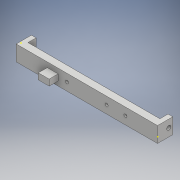
# Autodesk Inventor part: mtv_axelHolder(brakingAxel)3-12
Saved by Autodesk Inventor 2018 (Build 220112000, 112)
## iProperties
Created: 2019-03-12
Part Number: mtv_axelHolder(brakingAxel)3-12
Material: Generic
Document SubType Name: Sheet Metal
Designer: Aditya Kendre
Density: 1 g/cm^3
Sheet Metal Rule: Default_mm
Appearance: Default
Author: Aditya Kendre
Autodesk Inventor part; units mm, degrees
ref_plane "YZ Plane" through (0, 0, 0) normal (1, 0, 0) x (0, 1, 0)
ref_plane "XZ Plane" through (0, 0, 0) normal (0, 1, 0) x (-1, 0, 0)
ref_plane "XY Plane" through (0, 0, 0) normal (0, 0, 1) x (1, 0, 0)
sketch "Sketch1" plane through (0, 0, 0) normal (0, 1, 0) x (-1, 0, 0)
  line L0 (0, 0) -> (150, 0)
  line L1 (150, 0) -> (150, -19.925)
  line L2 (150, -19.925) -> (0, -19.925)
  line L3 (0, -19.925) -> (0, 0)
  dimension "d0" = 150
  dimension "d1" = 19.925
  constraints: 8 end point, 2 parallel, 1 horizontal, 1 perpendicular
  measures "d0" distance of L1.end L2.end
  measures "d1" distance of L0.end L1.end
extrude "Extrusion1" add sketch "Sketch1" along normal blind 4
sketch "Sketch2" plane through (0, 4, 0) normal (0, 1, 0) x (1, 0, 0)
  line L0 (-150, 0) -> (0, 0) projected
  line L1 (0, 19.925) -> (-150, 19.925) projected
  line L2 (0, 0) -> (-5, 0)
  line L3 (-5, 0) -> (-5, 19.925)
  line L4 (-5, 19.925) -> (0, 19.925)
  line L5 (0, 19.925) -> (0, 0)
  line L6 (-150.0001, 0) -> (-145.0001, 0)
  line L7 (-145.0001, 0) -> (-145.0001, 19.925)
  line L8 (-145.0001, 19.925) -> (-150.0001, 19.925)
  line L9 (-150.0001, 19.925) -> (-150.0001, 0)
  dimension "d4" = 5
  dimension "d5" = 5
  constraints: 16 end point, 4 parallel, 3 point on line, 2 horizontal, 2 perpendicular
  measures "d4" distance of L3.end L4.end
  measures "d5" distance of L8.end L7.end
extrude "Extrusion2" add sketch "Sketch2" along normal blind 12.175 contours L9 L1 L7 L0 | L3 L1 L5 L0
sketch "Sketch3" plane through (0, 4, 0) normal (0, 1, 0) x (1, 0, 0)
  line L0 (0, 19.925) -> (0, 0) projected
  line L1 (-150, 0) -> (-150, 19.925) projected
  line L2 (0, 19.925) -> (-150, 19.925)
  line L3 (-150, 19.925) -> (-150, 16.725)
  line L4 (-150, 16.725) -> (0, 16.725)
  line L5 (0, 16.725) -> (0, 19.925)
  dimension "d8" = 3.2
  constraints: 8 end point, 2 parallel, 1 horizontal, 1 perpendicular, 1 point on line
  measures "d8" distance of L3.end L2.end
extrude "Extrusion3" add sketch "Sketch3" along normal blind 4.65
sketch "Sketch4" plane through (0, 4, 0) normal (0, 1, 0) x (1, 0, 0)
  line L0 (-5, 16.725) -> (-145.0001, 16.725) construction
  line L1 (-145.0001, 0) -> (-145.0001, 19.925) construction
  line L2 (-5, 16.725) -> (-145.0001, 16.725) construction
  line L3 (-145.0001, 16.725) -> (-145.0001, 6.225) construction
  line L4 (-145.0001, 6.225) -> (-5, 6.225) construction
  line L5 (-5, 6.225) -> (-5, 16.725) construction
  line L6 (-5, 19.925) -> (-5, 0) projected
  line L7 (-145.0001, 6.225) -> (-5, 6.225)
  line L8 (-5, 6.225) -> (-5, 3.475)
  line L9 (-5, 3.475) -> (-145.0001, 3.475)
  line L10 (-145.0001, 3.475) -> (-145.0001, 6.225)
  point P0 (0, 0)
  dimension "d11" = 10.5
  dimension "d12" = 2.75
  constraints: 16 end point, 4 parallel, 2 horizontal, 2 perpendicular, 2 point on line
  measures "d11" distance of L3.end L2.end
  measures "d12" distance of L7.end L8.end
extrude "Extrusion4" add sketch "Sketch4" along normal blind 3.5
sketch "Sketch5" plane through (-145.0001, 4, 0) normal (1, 0, 0) x (0, 0, -1)
  point P0 (0, -4)
sketch "Sketch6" plane through (-145.0001, 4, 0) normal (1, 0, 0) x (0, 0, -1)
  line L0 (6.225, 0) -> (16.725, 0) construction
  line L1 (16.725, 0) -> (16.725, -7.95) construction
  line L2 (16.725, -7.95) -> (6.225, -7.95) construction
  line L3 (6.225, -7.95) -> (6.225, 0) construction
  line L4 (6.225, 0) -> (16.725, 0) construction
  line L5 (16.725, 0) -> (16.725, 7.95) construction
  line L6 (16.725, 7.95) -> (6.225, 7.95) construction
  line L7 (6.225, 7.95) -> (6.225, 0) construction
  circle A0 centre (11.475, 7.95) radius 2.25
  point P0 (0, -4)
  dimension "d15" = 7.95
  dimension "d16" = 7.95
  dimension "d17" = 4.5
  constraints: 16 end point, 4 parallel, 2 horizontal, 2 perpendicular, 1 centre point, 1 coincident, 1 midpoint, 1 point on line
  measures "d15" distance of L0.end L1.end
  measures "d16" distance of L5.end L4.end
  measures "d17" diameter of A0
extrude "Extrusion5" cut sketch "Sketch6" along normal blind 155.75 and the other way blind 5.75
sketch "Sketch7" plane through (0, 4, 0) normal (0, 1, 0) x (1, 0, 0)
  line L0 (-145.0001, 3.475) -> (-145.0001, 0) projected
  line L1 (-145.0001, 3.475) -> (1.5965, 3.475)
  line L2 (1.5965, 3.475) -> (1.5965, -1.1679)
  line L3 (1.5965, -1.1679) -> (-145.0001, -1.1679)
  line L4 (-145.0001, -1.1679) -> (-145.0001, 3.475)
  line L5 (-145.0001, 3.475) -> (-5, 3.475) projected
  line L6 (-145.0001, 3.475) -> (-155.2913, 3.475)
  line L7 (-155.2913, 3.475) -> (-155.2913, -7.4286)
  line L8 (-155.2913, -7.4286) -> (-145.0001, -7.4286)
  line L9 (-145.0001, -7.4286) -> (-145.0001, 3.475)
  point P0 (0, 0)
  constraints: 16 end point, 4 parallel, 2 horizontal, 2 perpendicular
extrude "Extrusion6" cut sketch "Sketch7" along normal blind 21 and the other way blind 34.875
sketch "Sketch8" plane through (0, 8.65, 0) normal (0, 1, 0) x (1, 0, 0)
  line L0 (-145.0001, 16.725) -> (-145.0001, 19.925) construction
  line L1 (-5, 16.725) -> (-145.0001, 16.725) construction
  line L2 (-145.0001, 19.925) -> (-5, 19.925) construction
  line L3 (-5, 19.925) -> (-5, 16.725) construction
  line L4 (-5, 16.725) -> (-145.0001, 16.725) construction
  line L5 (-145.0001, 16.725) -> (-145.0001, 19.925) construction
  line L6 (-150, 19.925) -> (0, 19.925) projected
  line L7 (-75, 19.925) -> (-70, 19.925)
  line L8 (-70, 19.925) -> (-70, 16.725)
  line L9 (-70, 16.725) -> (-75, 16.725)
  line L10 (-75, 16.725) -> (-75, 19.925)
  point P0 (0, 0)
  dimension "d26" = 5
  constraints: 16 end point, 4 parallel, 2 horizontal, 2 perpendicular, 1 midpoint, 1 point on line
  measures "d26" distance of L8.end L9.end
extrude "Extrusion7" add sketch "Sketch8" along normal blind 3.8
fillet "Fillet1" radius 3 1 edges at (-70, 12.45, -18.325)
fillet "Fillet2" radius 3 1 edges at (-70, 8.65, -18.325)
sketch "Sketch9" plane through (0, 4, 0) normal (0, 1, 0) x (1, 0, 0)
  line L0 (-145.0001, 13.725) -> (-145.0001, 9.225) construction
  line L1 (-5, 9.225) -> (-5, 13.725) construction
  line L2 (-75.0001, 11.475) -> (-96.0001, 11.475) construction
  circle A0 centre (-96.0001, 11.475) radius 1.65
  line L3 (-75.0001, 11.475) -> (-54.0001, 11.475) construction
  circle A1 centre (-54.0001, 11.475) radius 1.65
  point P0 (0, 0)
  dimension "d33" = 21
  dimension "d34" = 3.3
  dimension "d35" = 21
  dimension "d36" = 3.3
  constraints: 4 end point, 2 centre point, 2 coincident, 2 horizontal
  measures "d33" distance of L2.start L2.end
  measures "d34" diameter of A0
  measures "d35" distance of L2.start L3.end
  measures "d36" diameter of A1
extrude "Extrusion8" cut sketch "Sketch9" against normal blind 4
sketch "Sketch10" plane through (0, 4, 0) normal (0, 1, 0) x (1, 0, 0)
  circle A0 centre (-34, 11.475) radius 1.65 construction
  circle A1 centre (-34, 11.475) radius 1.65
  point P0 (0, 0)
  dimension "d39" = 3.3
  constraints: 2 centre point, 1 coincident, 1 concentric
  measures "d39" diameter of A0
extrude "Extrusion9" cut sketch "Sketch10" against normal blind 4
fillet "Fillet3" radius 2 3 edges at (-55.6501, 4, -11.475) (-35.65, 4, -11.475) (-97.6501, 4, -11.475)
sketch "Sketch11" plane through (0, 0, 0) normal (0, -1, 0) x (1, 0, 0)
  circle A0 centre (-96.0001, -11.475) radius 1.65 construction
  line L0 (-96.0001, -11.475) -> (-105.5001, -11.475) construction
  line L1 (-105.5, -8.75) -> (-105.5, -13.75)
  line L2 (-105.5, -13.75) -> (-117, -13.75)
  line L3 (-117, -13.75) -> (-117, -8.75)
  line L4 (-117, -8.75) -> (-105.5, -8.75)
  point P0 (0, 0)
  dimension "d43" = 9.5
  dimension "d44" = 5
  dimension "d45" = 11.5
  constraints: 10 end point, 2 parallel, 1 horizontal, 1 perpendicular, 1 vertical
  measures "d43" distance of L0.start L0.end
  measures "d44" distance of L1.start L1.end
  measures "d45" distance of L1.end L2.end
extrude "Extrusion10" add sketch "Sketch11" along normal blind 9.5
sketch "Sketch12" plane through (-105.5, 0, -13.75) normal (0, 0, -1) x (-1, 0, 0)
  line L0 (0, -9.5) -> (11.5, -9.5) construction
  line L1 (0, 0) -> (11.5, 0) construction
  line L2 (11.5, -9.5) -> (0, 0) construction
  line L3 (0, 0) -> (0, -9.5) construction
  line L4 (0, -9.5) -> (11.5, 0) construction
  circle A0 centre (5.75, -4.75) radius 2
  line L5 (11.5, -9.5) -> (0, -9.5)
  line L6 (0, -9.5) -> (0, 0)
  line L7 (0, 0) -> (11.5, 0)
  line L8 (11.5, 0) -> (11.5, -9.5)
  point P0 (-105.5, 0)
  dimension "d48" = 4
  constraints: 14 end point, 2 parallel, 2 perpendicular, 1 centre point, 1 horizontal, 1 midpoint
  measures "d48" diameter of A0
sketch "Sketch13" plane through (-105.5, 0, -13.75) normal (0, 0, -1) x (-1, 0, 0)
  point P0 (-105.5, 0)
extrude "Extrusion11" add sketch "Sketch12" along normal blind 1.5
sketch "Sketch14" plane through (-111.25, -4.75, -13.75) normal (0, 0, -1) x (-1, 0, 0)
  circle A0 centre (0, 0) radius 2
  point P0 (-111.25, 4.75)
  constraints: 1 centre point
extrude "Extrusion12" cut sketch "Sketch14" against normal blind 1.825
equation "\"BendRadius\" = Thickness"
equation "\"BendReliefWidth\" = Thickness"
equation "\"BendReliefDepth\" = 0.5 * Thickness"
equation "\"CornerReliefSize\" = 4 * Thickness"
equation "\"MinimumRemnant\" = 2 * Thickness"
equation "\"TransitionRadius\" = BendRadius"
equation "\"JacobiRadiusSize\" = BendRadius"
equation "\"GapSize\" = Thickness"
equation "\"Thickness\" = 0.5"
body "Solid1"
